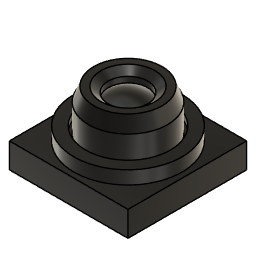
smart-sentry (Autodesk Fusion 360 archive; units mm, degrees)
design "OV3660"
Autodesk Fusion 360 part; units mm, degrees
sketch "Boceto1" plane through (0, 0, 0) normal (0, 0, 1) x (1, 0, 0)
  line L0 (-4.5, 4.5) -> (4.5, 4.5)
  line L1 (4.5, 4.5) -> (4.5, -4.5)
  line L2 (4.5, -4.5) -> (-4.5, -4.5)
  line L3 (-4.5, -4.5) -> (-4.5, 4.5)
  line L4 (-4.5, 0) -> (4.5, 0) construction
  circle A0 centre (0, 0) radius 4.1
  dimension "d1" = 9
  dimension "d3" = 8.2
  constraint horizontal L0
  constraint vertical L1
  constraint horizontal L2
  constraint vertical L3
  constraint equal L0 L1
  constraint midpoint L3 L4.start
  constraint midpoint L1 L4.end
  constraint midpoint A0.centre L4
  constraint coincident A0.centre origin
  measures "d1" distance of L0.start L0.end
  measures "d3" diameter of A0
extrude "Extruir1" add sketch "Boceto1" along normal blind 1.9 contours L0 L1 L2 L3 | A0
sketch "Boceto2" plane through (0, 0, 0) normal (0, 1, 0) x (1, 0, 0)
  line L0 (0, -5.0873) -> (0, 0)
  line L1 (-4.1, -1.9) -> (-4.1, -2.9)
  line L2 (-4.1, -2.9) -> (-3.2097, -2.9)
  line L3 (-3.2097, -2.9) -> (-3.2097, -2.4)
  line L4 (-3.2097, -2.4) -> (-3, -2.4)
  line L5 (-3, -2.4) -> (-3, -4.4695)
  line L6 (-3, -4.4695) -> (-2.5849, -5.5)
  line L7 (-2.5849, -5.5) -> (-2.0466, -5.5)
  line L8 (-4.1, -1.9) -> (0, -1.9)
  line L9 (-4.1, 0) -> (4.1, 0) construction
  line L10 (-2.0466, -5.5) -> (-1.5, -5.087)
  line L11 (-1.5, -5.087) -> (-1.5, -4.6497)
  arc A0 (-1.5, -4.6497) -> (0, -5.0873) centre (0, -2.2972) ccw
  line L12 (0, -5.0873) -> (0.6865, -5.0873) construction
  line L13 (0, -1.9) -> (0, -5.0873)
  dimension "d6" = 1.9
  dimension "d8" = 3.6
  dimension "d9" = 1
  dimension "d10" = 6
  dimension "d11" = 3
  constraint coincident L0.end origin
  constraint vertical L0
  constraint vertical L1
  constraint perpendicular L1 L2
  constraint perpendicular L2 L3
  constraint perpendicular L3 L4
  constraint perpendicular L4 L5
  constraint perpendicular L5 L7
  constraint coincident L0 L8.end
  constraint perpendicular L0 L8
  constraint coincident L1 L9.start
  constraint vertical L11
  constraint coincident L0 A0.end
  constraint tangent A0 L12
  constraint horizontal L12
  measures "d6" distance of L0.end L8
  measures "d8" distance of L7 L8
  measures "d9" distance of L1.start L1.end
revolve "Revolución1" add sketch "Boceto2" angle 360 about axis through (0, 0, 5.0873) along (0, 0, -1)

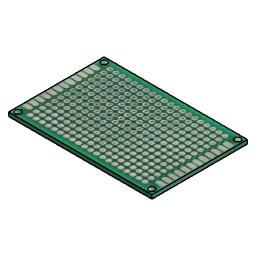
design "pcb"
Autodesk Fusion 360 part; units mm, degrees
sketch "Boceto1" plane through (0, 0, 0) normal (0, 0, 1) x (1, 0, 0)
  line L0 (-30, 20) -> (30, 20)
  line L1 (30, 20) -> (30, -20)
  line L2 (30, -20) -> (-30, -20)
  line L3 (-30, -20) -> (-30, 20)
  line L4 (-30, 0) -> (30, 0) construction
  circle A0 centre (28, -18) radius 1.27
  line L5 (0, 0) -> (0, -20) construction
  circle A1 centre (-28, -18) radius 1.27
  circle A2 centre (28, 18) radius 1.27
  circle A3 centre (-28, 18) radius 1.27
  dimension "d1" = 40
  dimension "d2" = 60
  dimension "d5" = 2.54
  dimension "d6" = 56
  dimension "d7" = 36
  constraint horizontal L0
  constraint vertical L1
  constraint horizontal L2
  constraint vertical L3
  constraint coincident L3 L4.start
  constraint coincident L1 L4.end
  constraint perpendicular L1 L4
  constraint midpoint L5.start L4
  constraint midpoint L3 L4.start
  constraint coincident L5.start origin
  constraint midpoint L2 L5.end
  constraint symmetric A0 L5 A1
  constraint symmetric L4 A0 A2
  constraint symmetric L4 A1 A3
  measures "d1" distance of L0.start L2.end
  measures "d2" distance of L0.start L0.end
  measures "d5" diameter of A0
  measures "d6" distance of A0.centre A1.centre
  measures "d7" distance of A0.centre A2.centre
extrude "Extruir1" add sketch "Boceto1" along normal blind 1.6

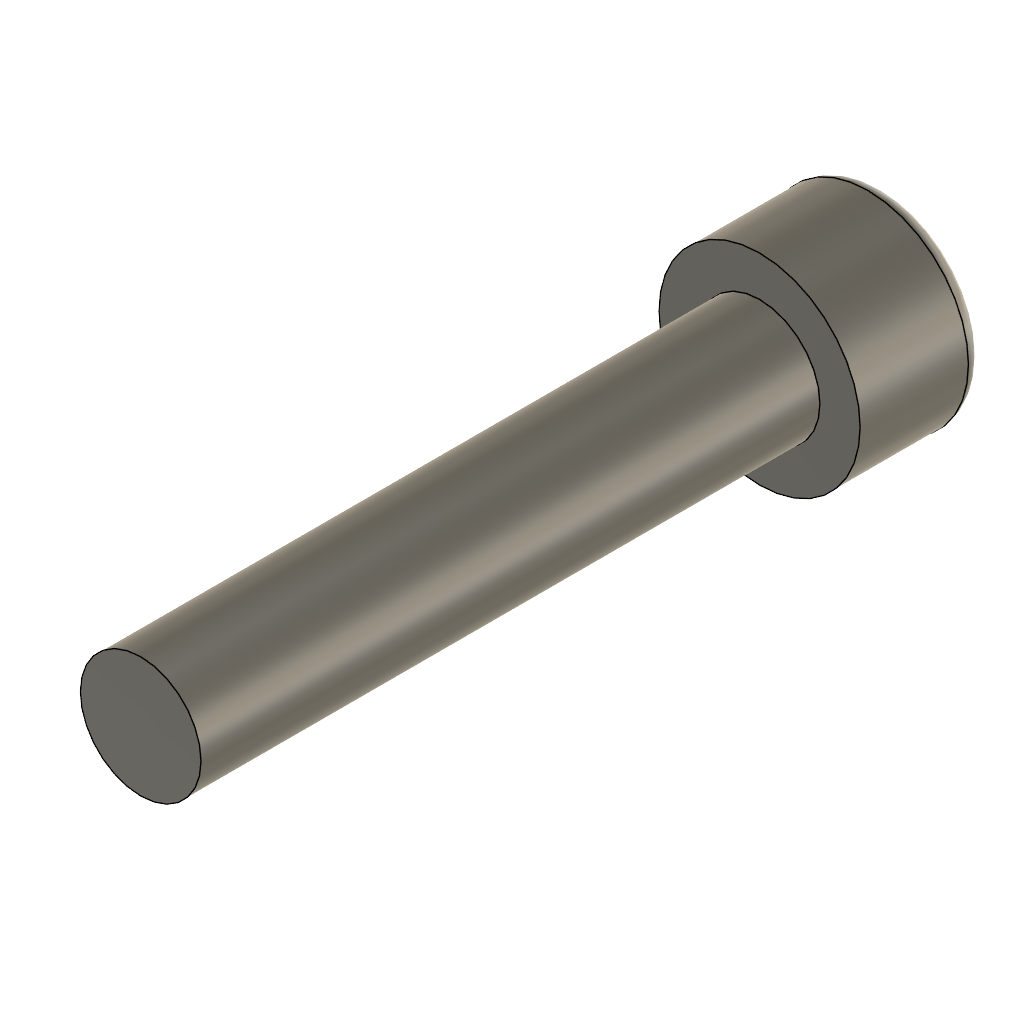
design "M8-40 allen"
Autodesk Fusion 360 part; units mm, degrees
sketch "Boceto1" plane through (0, 0, 0) normal (0, 0, 1) x (1, 0, 0)
  line L0 (0, 8) -> (-6.5, 8)
  line L1 (-6.5, 8) -> (-6.5, 0)
  line L2 (-6.5, 0) -> (-3.9, 0)
  line L3 (-3.9, 0) -> (-3.9, -40)
  line L4 (-3.9, -40) -> (0, -40)
  line L5 (0, -40) -> (0, 8)
  dimension "d1" = 7.8
  dimension "d2" = 13
  dimension "d3" = 8
  dimension "d4" = 40
  constraint horizontal L0
  constraint perpendicular L0 L1
  constraint perpendicular L1 L2
  constraint perpendicular L0 L3
  constraint perpendicular L1 L4
  constraint coincident origin L2
  constraint coincident origin L5
  constraint vertical L5
  measures "d3" distance of L0.end L1.end
  measures "d4" distance of L2.end L3.end
revolve "Revolución1" add sketch "Boceto1" angle 360 about axis through (0, -40, 0) along (0, 1, 0)
sketch "Boceto2" plane through (0, 0, 0) normal (0, 1, 0) x (1, 0, 0)
  line L0 (1.7321, 3) -> (-1.7321, 3)
  line L1 (-1.7321, 3) -> (-3.4641, 0)
  line L2 (-3.4641, 0) -> (-1.7321, -3)
  line L3 (-1.7321, -3) -> (1.7321, -3)
  line L4 (1.7321, -3) -> (3.4641, 0)
  line L5 (3.4641, 0) -> (1.7321, 3)
  dimension "d6" = 6
  constraint horizontal L0
  measures "d6" distance of L1 L4
extrude "Extruir1" cut sketch "Boceto2" along normal through all from surface at 3
fillet "Empalme1" radius 1 1 edges at (-6.0601, 8, 2.3505)

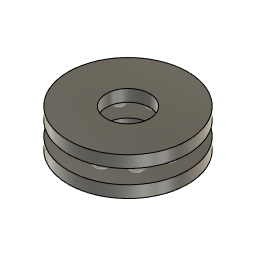
design "bearing axial"
Autodesk Fusion 360 part; units mm, degrees
sketch "Sketch1" plane through (0, 0, 0) normal (0, 1, 0) x (1, 0, 0)
  line L0 (-4, -7) -> (-11, -7)
  line L1 (-11, -7) -> (-11, -4.8)
  line L2 (-11, -4.8) -> (-4, -4.8)
  line L3 (-4, -4.8) -> (-4, -7)
  line L4 (-11, -2.2) -> (-4.1, -2.2)
  line L5 (-4.1, -2.2) -> (-4.1, 0)
  line L6 (-4.1, 0) -> (-11, 0)
  line L7 (-11, 0) -> (-11, -2.2)
  circle A0 centre (-7.5, -3.5) radius 1.6
  line L8 (0, 0) -> (0, -64)
  line L9 (-7.5, 0) -> (-7.5, -7) construction
  dimension "d13" = 3.2
  dimension "d14" = 2.2
  dimension "d15" = 22
  dimension "d16" = 8
  dimension "d17" = 8.2
  dimension "d18" = 7
  constraint horizontal L0
  constraint vertical L1
  constraint horizontal L2
  constraint vertical L3
  constraint horizontal L4
  constraint vertical L5
  constraint horizontal L6
  constraint vertical L7
  constraint equal L1 L7
  constraint coincident L8.start origin
  constraint perpendicular L6 L8
  constraint vertical L1.end L4.start
  constraint midpoint L0 L9.end
  constraint vertical L9
  constraint midpoint A0.centre L9
  constraint coincident L6 L9.start
  constraint horizontal L8.start L5.end
  measures "d13" diameter of A0
  measures "d14" distance of L0.end L1.end
  measures "d18" distance of L0 L6
revolve "Revolve2" add sketch "Sketch1" angle 360 about axis through (0, 0, 0) along (0, 0, 1) contours L0 L1 L2 L3 A0 | L2 A0 | L4 A0 | L4 L5 L6 L7 A0 makes body 1 at (-8.6438, 0.7502, 2.2) makes body 2 at (-8.6257, 0.5465, 7)
sketch "Sketch2" plane through (0, 0, 0) normal (0, 1, 0) x (1, 0, 0)
  line L0 (-7.5, 0) -> (-7.5, -7)
  arc A0 (-7.5, -1.9) -> (-7.5, -5.1) centre (-7.5, -3.5) ccw
  point P0 (-7.5, -3.5)
  point P1 (-7.5, 0)
  point P2 (-7.5, -7)
  constraint coincident P0 A0.centre
  constraint coincident P1 L0.start
  constraint coincident P2 L0.end
  constraint coincident L0 A0.end
  constraint coincident L0 A0.start
revolve "Revolve3" add sketch "Sketch2" angle 360 about axis through (-7.5, 0, 0) along (0, 0, 1) separate body makes body 3
pattern_circular "C-Pattern1" count 10 over 360 about axis through (0, 0, 0) along (0, 0, 1) of bodies 3 makes body 4 at (-7.0725, -5.606, 3.1595) makes body 5 at (-2.4267, -8.6925, 3.1595) makes body 6 at (3.1461, -8.4587, 3.1595) makes body 7 at (7.5171, -4.994, 3.1595) makes body 8 at (9.0169, 0.3782, 3.1595) makes body 9 at (7.0725, 5.606, 3.1595) makes body 10 at (2.4267, 8.6925, 3.1595) makes body 11 at (-3.1461, 8.4587, 3.1595) makes body 12 at (-7.5171, 4.994, 3.1595)

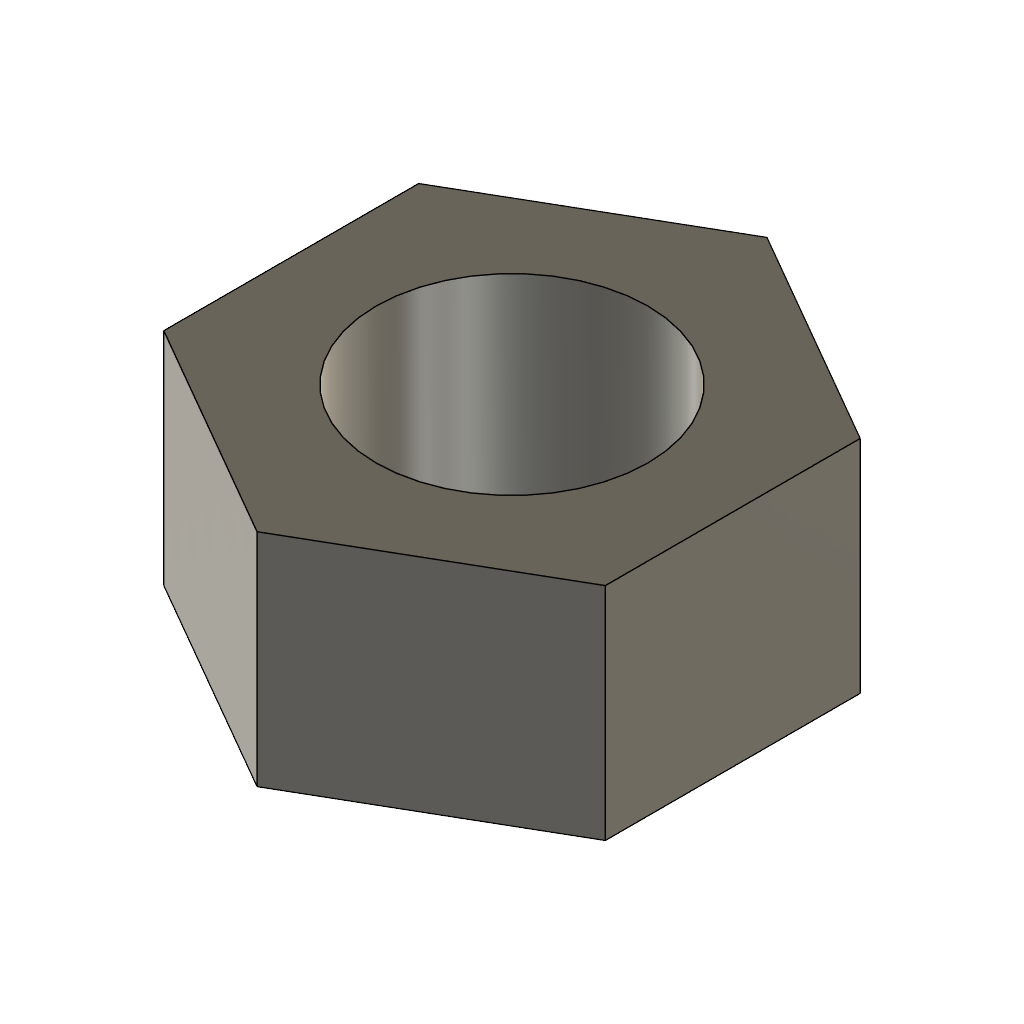
design "tuerca M8"
Autodesk Fusion 360 part; units mm, degrees
sketch "Boceto1" plane through (0, 0, 0) normal (0, 0, 1) x (1, 0, 0)
  line L0 (6.5, 3.7528) -> (0, 7.5056)
  line L1 (0, 7.5056) -> (-6.5, 3.7528)
  line L2 (-6.5, 3.7528) -> (-6.5, -3.7528)
  line L3 (-6.5, -3.7528) -> (0, -7.5056)
  line L4 (0, -7.5056) -> (6.5, -3.7528)
  line L5 (6.5, -3.7528) -> (6.5, 3.7528)
  circle A0 centre (0, 0) radius 4
  dimension "d1" = 13
  dimension "d2" = 8
  constraint coincident A0.centre origin
  constraint vertical L2
  measures "d1" distance of L2 L5
  measures "d2" diameter of A0
extrude "Extruir1" add sketch "Boceto1" along normal blind 6.5

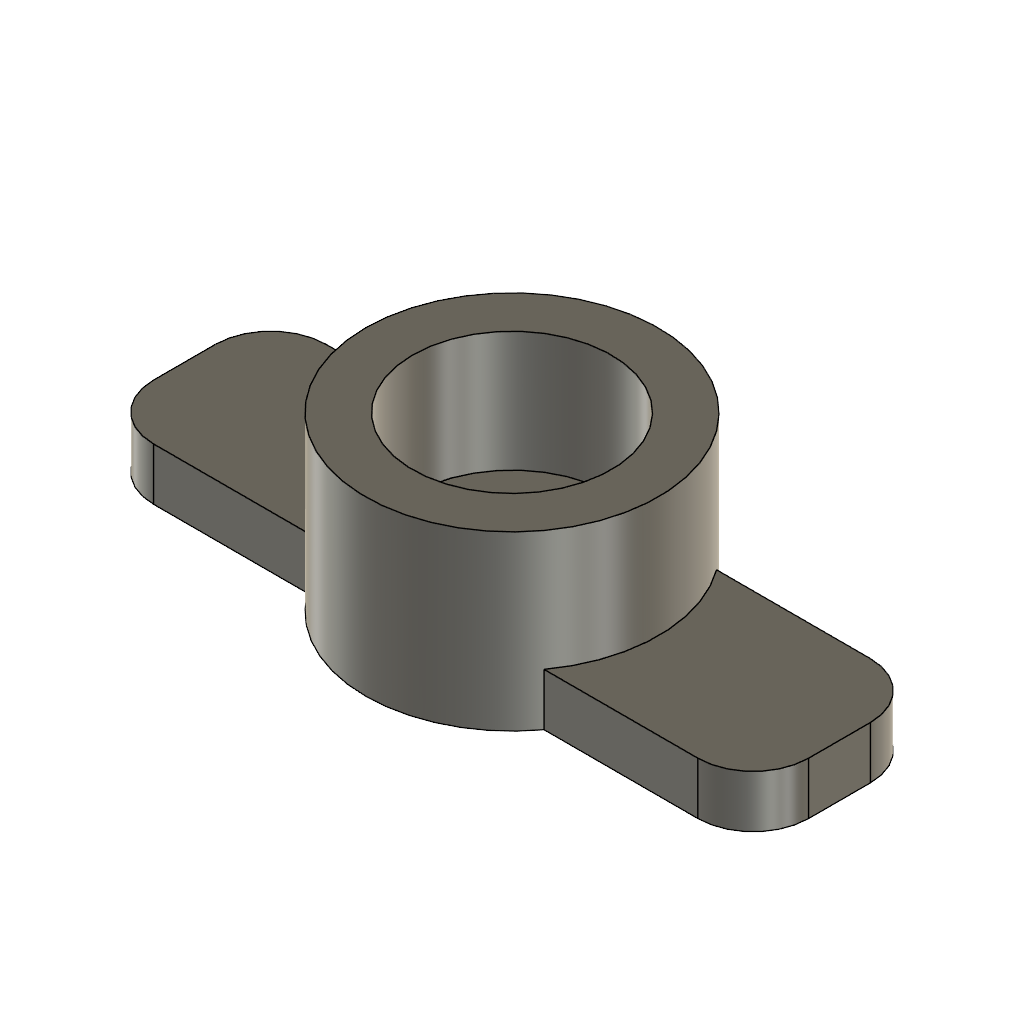
design "horn"
Autodesk Fusion 360 part; units mm, degrees
sketch "Boceto1" plane through (0, 0, 0) normal (0, 0, 1) x (1, 0, 0)
  circle A0 centre (0, 0) radius 2.8
  line L0 (-6.2622, 1.65) -> (6.2622, 1.65)
  line L1 (6.2622, 1.65) -> (6.2622, -1.65)
  line L2 (6.2622, -1.65) -> (-6.2622, -1.65)
  line L3 (-6.2622, -1.65) -> (-6.2622, 1.65)
  line L4 (-6.2622, 0) -> (6.2622, 0) construction
  line L5 (0, 1.65) -> (0, 0) construction
  circle A1 centre (0, 0) radius 0.75
  circle A2 centre (0, 0) radius 1.9
  point P0 (2.2622, 1.65)
  dimension "d1" = 5.6
  dimension "d2" = 3.3
  dimension "d3" = 4
  dimension "d8" = 1.5
  dimension "d9" = 3.8
  constraint coincident A0.centre L5.end
  constraint horizontal L0
  constraint vertical L1
  constraint horizontal L2
  constraint vertical L3
  constraint midpoint L3 L4.start
  constraint midpoint L1 L4.end
  constraint midpoint L0 L5.start
  constraint midpoint L4 A0.centre
  constraint coincident A0 P0
  constraint coincident L0 P0
  measures "d1" diameter of A0
  measures "d2" distance of L0 L2
  measures "d3" distance of L1 P0
  measures "d8" diameter of A1
  measures "d9" diameter of A2
extrude "Extruir1" add sketch "Boceto1" along normal blind 1 contours A0 L0 L2 A2 | A0 L0 L1 L2 | A0 L0 L2 A2 | A0 L0 L2 L3 | L0 L2 A2
extrude "Extruir2" add sketch "Boceto1" along normal blind 3.3 contours A0 L0 L2 A2 | A0 L0 A2 | A0 L2 A2 | A0 L0 L2 A2 | L0 L2 A2 | L0 A2 | L2 A2
extrude "Extruir3" cut sketch "Boceto1" along normal through all from surface at 1 contours L0 L2 A2 | L0 A2 | L2 A2
fillet "Empalme1" radius 1.059 4 edges at (-6.2622, 1.65, 0.5) (-6.2622, -1.65, 0.5) (6.2622, 1.65, 0.5) (6.2622, -1.65, 0.5)
